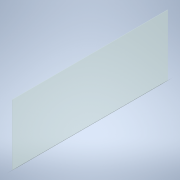
# Autodesk Inventor part: glass_slab
Saved by Autodesk Inventor 2020 (Build 240168000, 168)
## iProperties
Created: 2020-04-13
Part Number: glass_slab
Material: Glass
Document SubType Name: Modeling
Designer: LENOVO
Density: 2.18 g/cm^3
Appearance: Clear
Author: LENOVO
Autodesk Inventor part; units mm, degrees
ref_plane "YZ Plane" through (0, 0, 0) normal (1, 0, 0) x (0, 1, 0)
ref_plane "XZ Plane" through (0, 0, 0) normal (0, 1, 0) x (-1, 0, 0)
ref_plane "XY Plane" through (0, 0, 0) normal (0, 0, 1) x (1, 0, 0)
sketch "Sketch1" plane through (0, 0, 0) normal (1, 0, 0) x (0, 1, 0)
  line L0 (195, 495) -> (-195, 495)
  line L1 (-195, 495) -> (-195, -495)
  line L2 (-195, -495) -> (195, -495)
  line L3 (195, -495) -> (195, 495)
  line L4 (195, 495) -> (-195, -495) construction
  line L5 (-195, 495) -> (195, -495) construction
  point P0 (0, 0)
  dimension "d0" = 390
  dimension "d1" = 990
  constraints: 12 end point, 2 midpoint, 2 parallel, 1 horizontal, 1 perpendicular
  measures "d0" distance of L2.end L1.end
  measures "d1" distance of L1.end L0.end
extrude "Extrusion1" add sketch "Sketch1" along normal blind 2
body "Solid1"
